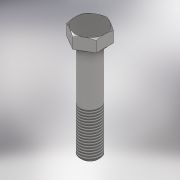
# Autodesk Inventor part: Part16 Real Bolt Thread
Saved by Autodesk Inventor 2022.2 (Build 262287010, 287A)
## iProperties
Created: 2022-12-19
Part Number: Part16 Real Bolt Thread
Material: Steel
Document SubType Name: Modeling
Designer: User
Mass: 527.789 g
Surface Area: 152.44 cm^2
Volume: 67.2343 cm^3
Density: 7.85 g/cm^3
Appearance: Semi-Polished
Author: User
Autodesk Inventor part; units mm, degrees
ref_plane "YZ Plane" through (0, 0, 0) normal (1, 0, 0) x (0, 1, 0)
ref_plane "XZ Plane" through (0, 0, 0) normal (0, 1, 0) x (-1, 0, 0)
ref_plane "XY Plane" through (0, 0, 0) normal (0, 0, 1) x (1, 0, 0)
sketch "Sketch1" plane through (0, 0, 0) normal (0, 1, 0) x (-1, 0, 0)
  line L0 (127.8939, 73.8396) -> (127.8939, -73.8396)
  line L1 (127.8939, -73.8396) -> (0, -147.6791)
  line L2 (0, -147.6791) -> (-127.8939, -73.8396)
  line L3 (-127.8939, -73.8396) -> (-127.8939, 73.8396)
  line L4 (-127.8939, 73.8396) -> (0, 147.6791)
  line L5 (0, 147.6791) -> (127.8939, 73.8396)
  line L6 (-18, 10.3923) -> (0, 20.7846)
  line L7 (0, 20.7846) -> (18, 10.3923)
  line L8 (18, 10.3923) -> (18, -10.3923)
  line L9 (18, -10.3923) -> (0, -20.7846)
  line L10 (0, -20.7846) -> (-18, -10.3923)
  line L11 (-18, -10.3923) -> (-18, 10.3923)
  point P0 (0, 0)
  point P1 (0, 0)
  point P2 (0, 0)
  dimension "Shex" = 36
  constraints: 24 end point, 2 coincident, 2 vertical, 26 other
  measures "Shex" distance between parallel lines of L11 L8
extrude "Extrusion1" add sketch "Sketch1" along normal blind 15 contours L6 L7 L8 L9 L10 L11
sketch "Sketch2" plane through (0, 0, 0) normal (1, 0, 0) x (0, 1, 0)
  line L0 (0, -20.7846) -> (15, -20.7846) construction
  line L1 (15, -20.7846) -> (13.3923, -20.7846)
  line L2 (13.3923, -20.7846) -> (15, -18)
  line L3 (15, -18) -> (15, -20.7846)
  line L4 (-3, 0) -> (18, 0) projected
  point P0 (0, 0)
  dimension "d4" = 60
  dimension "d5" = 36
  constraints: 6 end point, 1 point on line, 1 vertical
  measures "d4" angle of L2 L0
  measures "d5" diameter of L2.end L4
revolve "Revolution1" cut sketch "Sketch2" angle 360 about axis through (0, -10, 0) along (0, 1, 0)
sketch "Sketch3" plane through (0, 0, 0) normal (0, 0, 1) x (1, 0, 0)
  line L0 (0, 0) -> (12, 0)
  line L1 (12, 0) -> (12, -120)
  line L2 (12, -120) -> (0, -120)
  line L3 (0, -120) -> (0, 0)
  dimension "L" = 120
  dimension "Dia" = 24
  constraints: 8 end point, 2 parallel, 1 horizontal, 1 perpendicular
  measures "L" distance of L0.end L1.end
  measures "Dia" diameter of L1 L3
revolve "Revolution2" add sketch "Sketch3" angle 360 about axis through (0, -120, 0) along (0, 1, 0)
fillet "Fillet1" radius 0.8 1 edges at (-12, 0, 0)
chamfer "Chamfer1" distance 2 angle 45 1 edges at (-12, -120, 0)
thread "Thread2" size "M24x3" class "6g" standard "ANSI Metric M Profile" length 54
sketch "Sketch6" plane through (0, 0, 0) normal (1, 0, 0) x (0, 1, 0)
  line L0 (-147, 0) -> (42, 0) projected
  line L1 (0, -20.7846) -> (13.3923, -20.7846) projected
  line L2 (0, -20.7846) -> (0, -10.3923) projected
  line L3 (0, -10.3923) -> (13.3923, -10.3923) projected
  line L4 (0, -20.7846) -> (0.5, -20.7846)
  line L5 (0.5, -20.7846) -> (0.5, -18)
  line L6 (0.5, -18) -> (0, -18)
  line L7 (0, -18) -> (0, -20.7846)
  point P0 (0, 0)
  point P1 (15, -15.5885)
  point P2 (0, -18)
  dimension "a" = 0.5
  dimension "d34" = 36
  constraints: 8 end point, 2 parallel, 1 horizontal, 1 perpendicular, 2 other
  measures "a" distance of L6.end L5.end
  measures "d34" diameter of L6 L0
revolve "Revolution3" cut sketch "Sketch6" angle 360 about axis through (0, -10, 0) along (0, 1, 0)
equation "\"d5\" = Shex"
equation "\"d31\" = b - cham"
equation "\"d34\" = Shex"
equation "\"b\" = 56"
equation "\"cham\" = 2"
body "Solid1"
